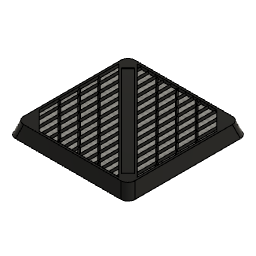
Air filter 120mm (Autodesk Fusion 360 design; units mm, degrees)
Autodesk Fusion 360 part; units mm, degrees
ref_plane "WorkPlane3" through (0, -60, 0) normal (0, 1, 0) x (0, 0, 1)
sketch "Frame bars" plane through (0, -60, 0) normal (0, 1, 0) x (1, 0, 0)
  line L0 (0, 0) -> (0, -95) construction
  line L1 (-60, 0) -> (-60, -25) construction
  line L2 (-52, 0) -> (-52, -10) construction
  line L3 (-44, 0) -> (-44, -10) construction
  line L4 (-36, 0) -> (-36, -10) construction
  line L5 (-28, 0) -> (-28, -10) construction
  line L6 (-20, 0) -> (-20, -10) construction
  line L7 (-12, 0) -> (-12, -10) construction
  line L8 (-4, 0) -> (-4, -10) construction
  line L9 (4, 0) -> (4, -10) construction
  line L10 (12, 0) -> (12, -10) construction
  line L11 (20, 0) -> (20, -10) construction
  line L12 (28, 0) -> (28, -10) construction
  line L13 (36, 0) -> (36, -10) construction
  line L14 (44, 0) -> (44, -10) construction
  line L15 (-63, -2) -> (49, -2) construction
  line L16 (0, 0) -> (49, 0) construction
  line L17 (-61, 0) -> (-60, -2)
  line L18 (-60, -2) -> (-59, 0)
  line L19 (-59, 0) -> (-61, 0)
  line L20 (-51, 0) -> (-53, 0)
  line L21 (-53, 0) -> (-52, -2)
  line L22 (-52, -2) -> (-51, 0)
  line L23 (-45, 0) -> (-44, -2)
  line L24 (-44, -2) -> (-43, 0)
  line L25 (-43, 0) -> (-45, 0)
  line L26 (-37, 0) -> (-36, -2)
  line L27 (-36, -2) -> (-35, 0)
  line L28 (-35, 0) -> (-37, 0)
  line L29 (-29, 0) -> (-28, -2)
  line L30 (-28, -2) -> (-27, 0)
  line L31 (-27, 0) -> (-29, 0)
  line L32 (-21, 0) -> (-20, -2)
  line L33 (-20, -2) -> (-19, 0)
  line L34 (-19, 0) -> (-21, 0)
  line L35 (-13, 0) -> (-12, -2)
  line L36 (-12, -2) -> (-11, 0)
  line L37 (-11, 0) -> (-13, 0)
  line L38 (-5, 0) -> (-4, -2)
  line L39 (-4, -2) -> (-3, 0)
  line L40 (-3, 0) -> (-5, 0)
  line L41 (3, 0) -> (4, -2)
  line L42 (4, -2) -> (5, 0)
  line L43 (11, 0) -> (12, -2)
  line L44 (12, -2) -> (13, 0)
  line L45 (20, -2) -> (21, 0)
  line L46 (19, 0) -> (20, -2)
  line L47 (28, -2) -> (29, 0)
  line L48 (27, 0) -> (28, -2)
  line L49 (36, -2) -> (37, 0)
  line L50 (35, 0) -> (36, -2)
  line L51 (44, -2) -> (45, 0)
  line L52 (43, 0) -> (44, -2)
  line L53 (5, 0) -> (3, 0)
  line L54 (13, 0) -> (11, 0)
  line L55 (21, 0) -> (19, 0)
  line L56 (29, 0) -> (27, 0)
  line L57 (37, 0) -> (35, 0)
  line L58 (45, 0) -> (43, 0)
  dimension "d1" = 60
  dimension "d2" = 8
  dimension "d3" = 8
  dimension "d4" = 8
  dimension "d5" = 8
  dimension "d6" = 8
  dimension "d7" = 8
  dimension "d8" = 8
  dimension "d9" = 8
  dimension "d10" = 8
  dimension "d11" = 8
  dimension "d12" = 8
  dimension "d13" = 8
  dimension "d14" = 8
  dimension "d15" = 2
  constraint coincident L0.start L16.start
  constraint vertical L0
  constraint vertical L1
  constraint vertical L2
  constraint vertical L3
  constraint vertical L4
  constraint vertical L5
  constraint vertical L6
  constraint vertical L7
  constraint vertical L8
  constraint vertical L9
  constraint vertical L10
  constraint vertical L11
  constraint vertical L12
  constraint parallel L12 L13
  constraint vertical L14
  constraint perpendicular L13 L15
  constraint perpendicular L14 L16
  constraint coincident L15 L17.end
  constraint coincident L1 L17.end
  constraint parallel L15 L19
  constraint perpendicular L2 L20
  constraint coincident L15 L21.end
  constraint coincident L2 L21.end
  constraint coincident L3 L23.end
  constraint coincident L15 L23.end
  constraint parallel L21 L23
  constraint parallel L22 L24
  constraint perpendicular L3 L25
  constraint coincident L4 L26.end
  constraint coincident L15 L26.end
  constraint parallel L24 L27
  constraint perpendicular L4 L28
  constraint coincident L15 L29.end
  constraint coincident L5 L29.end
  constraint parallel L27 L30
  constraint perpendicular L5 L31
  constraint coincident L6 L32.end
  constraint coincident L15 L32.end
  constraint parallel L30 L33
  constraint perpendicular L6 L34
  constraint coincident L7 L35.end
  constraint coincident L15 L35.end
  constraint parallel L33 L36
  constraint perpendicular L7 L37
  constraint coincident L8 L38.end
  constraint coincident L15 L38.end
  constraint parallel L36 L39
  constraint perpendicular L8 L40
  constraint coincident L16 L41.start
  constraint coincident L15 L41.end
  constraint parallel L38 L41
  constraint coincident L16 L42.end
  constraint parallel L39 L42
  constraint coincident L16 L43.start
  constraint coincident L15 L43.end
  constraint coincident L10 L43.end
  constraint coincident L16 L44.end
  constraint coincident L15 L45.start
  constraint coincident L11 L45.start
  constraint coincident L16 L45.end
  constraint coincident L16 L46.start
  constraint coincident L15 L47.start
  constraint coincident L12 L47.start
  constraint coincident L16 L47.end
  constraint parallel L45 L47
  constraint coincident L16 L48.start
  constraint parallel L46 L48
  constraint coincident L15 L49.start
  constraint coincident L13 L49.start
  constraint coincident L16 L49.end
  constraint parallel L47 L49
  constraint coincident L16 L50.start
  constraint parallel L48 L50
  constraint coincident L15 L51.start
  constraint coincident L14 L51.start
  constraint coincident L16 L51.end
  constraint parallel L49 L51
  constraint coincident L16 L52.start
  constraint parallel L50 L52
  measures "d1" distance of L0 L1
  measures "d2" distance of L1 L2
  measures "d3" distance of L2 L3
  measures "d4" distance of L3 L4
  measures "d5" distance of L4 L5
  measures "d6" distance of L5 L6
  measures "d7" distance of L6 L7
  measures "d8" distance of L7 L8
  measures "d9" distance of L8 L9
  measures "d10" distance of L9 L10
  measures "d11" distance of L10 L11
  measures "d12" distance of L11 L12
  measures "d13" distance of L12 L13
  measures "d14" distance of L13 L14
  measures "d15" distance of L15 L16
  measures "d95" distance of L0.start
  measures "d103" distance of L0.start
  measures "d104" distance of L0.start
sketch "Frame Edge" plane through (0, 0, 0) normal (0, 0, 1) x (1, 0, 0)
  line L0 (0, 0) -> (0, 72.5) construction
  line L1 (0, 0) -> (90, 0) construction
  circle A0 centre (-52.5, 52.5) radius 2.75
  circle A1 centre (-52.5, -52.5) radius 2.75
  circle A2 centre (52.5, 52.5) radius 2.75
  circle A3 centre (52.5, -52.5) radius 2.75
  line L2 (-57.4497, 47.5503) -> (47.5503, -57.4497)
  arc A4 (47.5503, -57.4497) -> (57.4497, -47.5503) centre (52.5, -52.5) ccw
  line L3 (57.4497, -47.5503) -> (-47.5503, 57.4497)
  arc A5 (-47.5503, 57.4497) -> (-57.4497, 47.5503) centre (-52.5, 52.5) ccw
  line L4 (-52.5, 52.5) -> (52.5, -52.5) construction
  circle A6 centre (-52.5, -52.5) radius 7
  circle A7 centre (52.5, 52.5) radius 7
  line L5 (59.5, 52.5) -> (59.5, -52.5)
  line L6 (-59.5, 52.5) -> (-59.5, -52.5)
  line L7 (52.5, 59.5) -> (-52.5, 59.5)
  line L8 (52.5, -59.5) -> (-52.5, -59.5)
  line L9 (35.5, 59.5) -> (59.5, 35.5)
  line L10 (35.5, 59.5) -> (69.5744, 59.5) construction
  line L11 (-59.5, -35.5) -> (-35.5, -59.5)
  line L12 (-52.5, 57.5) -> (52.5, 57.5)
  line L13 (-53.8563, -57.5) -> (52.5, -57.5)
  line L14 (-53.9142, 44.0147) -> (-52.5, 45.4289) construction
  line L15 (-52.5, 45.4289) -> (-44.0147, 53.9142) construction
  line L16 (44.0147, -53.9142) -> (53.9142, -44.0147) construction
  line L17 (-52.5, 45.4289) -> (45.4289, -52.5)
  line L18 (45.4289, -52.5) -> (52.5, -45.4289)
  line L19 (52.5, -45.4289) -> (-45.4289, 52.5)
  line L20 (-45.4289, 52.5) -> (-52.5, 45.4289)
  line L21 (-57.5, -52.5) -> (-57.5, 52.5)
  line L22 (57.5, -52.5) -> (57.5, 52.5)
  circle A8 centre (-52.5, -52.5) radius 5
  circle A9 centre (-52.5, 52.5) radius 5
  circle A10 centre (52.5, -52.5) radius 5
  circle A11 centre (52.5, 52.5) radius 5
  circle A12 centre (-52.5, 52.5) radius 4
  circle A13 centre (-52.5, -52.5) radius 4
  circle A14 centre (52.5, 52.5) radius 4
  circle A15 centre (52.5, -52.5) radius 4
  dimension "d19" = 5.5
  dimension "d20" = 52.5
  dimension "d21" = 52.5
  dimension "d22" = 14
  dimension "d23" = 14
  dimension "d24" = 14
  dimension "d25" = 45
  dimension "d26" = 24
  dimension "d27" = 2
  dimension "d28" = 2
  dimension "d29" = 5
  dimension "d30" = 5
  dimension "d31" = 2
  dimension "d32" = 2
  dimension "d33" = 2
  dimension "d117" = 10
  dimension "d118" = 8
  constraint coincident L0.start L1.start
  constraint vertical L0
  constraint perpendicular L0 L1
  constraint symmetric L1 A0 A1
  constraint symmetric L0 A0 A2
  constraint symmetric L0 A1 A3
  constraint tangent L2 A4
  constraint tangent A4 L3
  constraint parallel L2 L3
  constraint tangent L3 A5
  constraint tangent L2 A5
  constraint coincident A3.centre A4.centre
  constraint coincident A0.centre A5.centre
  constraint concentric A1 A6
  constraint concentric A2 A7
  constraint coincident A7 L5.start
  constraint coincident A4 L5.end
  constraint tangent A4 L5
  constraint tangent A7 L5
  constraint symmetric L0 L5.start L6.start
  constraint symmetric L0 L5.end L6.end
  constraint coincident A7 L7.start
  constraint coincident A5 L7.end
  constraint tangent A5 L7
  constraint tangent A7 L7
  constraint symmetric L1 L7.start L8.start
  constraint symmetric L1 L7.end L8.end
  constraint horizontal L10
  constraint coincident L7 L9.start
  constraint coincident L5 L9.end
  constraint symmetric L4 L9.start L11.start
  constraint symmetric L4 L9.end L11.end
  constraint perpendicular L0 L12
  constraint horizontal L13
  constraint perpendicular L4 L14
  constraint perpendicular L4 L15
  constraint perpendicular L4 L16
  constraint coincident L3 L16.end
  constraint coincident L2 L16.start
  constraint coincident L3 L15.end
  constraint coincident L2 L14.start
  constraint perpendicular L17 L18
  constraint parallel L17 L19
  constraint parallel L18 L20
  constraint coincident L16 L17.end
  constraint perpendicular L16 L17
  constraint vertical L21
  constraint symmetric L0 L21.start L22.start
  constraint symmetric L0 L21.end L22.end
  constraint concentric A1 A8
  constraint symmetric L1 A8 A9
  constraint symmetric L0 A8 A10
  constraint symmetric L0 A9 A11
  constraint coincident L13.end A10
  constraint coincident L21.start A8
  constraint coincident L21.end A9
  constraint coincident L12.start A9
  constraint coincident L12.end A11
  constraint concentric A0 A12
  constraint symmetric L1 A12 A13
  constraint symmetric L0 A12 A14
  constraint symmetric L0 A13 A15
  measures "d19" diameter of A0
  measures "d20" distance of L0 A0.centre
  measures "d21" distance of L1 A0.centre
  measures "d22" diameter of A4
  measures "d23" diameter of A6
  measures "d24" diameter of A7
  measures "d25" angle of L9 L10
  measures "d26" distance of L5 L9.start
  measures "d27" distance of L7 L12
  measures "d28" distance of L8 L13
  measures "d29" distance of A0.centre L15
  measures "d30" distance of A3.centre L16
  measures "d31" distance of L2 L17
  measures "d32" distance of L3 L19
  measures "d33" distance of L6 L21
  measures "d117" diameter of A8
  measures "d118" diameter of A12
extrude "Extrude1" add sketch "Frame Edge" along normal blind 3 contours L2 A4 A5 L13 L17 L18 L20 L21 A9 A10 | A5 L6 L11 L21 | A5 L12 L21 A9 | A4 L13 L22 A10 | A4 L8 L11 L13 | A6 L6 L11 L21 | A6 L11 L13 L21 | A9 | A6 L8 L11 L13 | A10 | A5 L7 L9 L12 | A6 L13 L21 A8 | A6 L13 L21 A8 | A4 L3 A5 L12 L18 L19 L20 L22 A9 A10 | A4 L5 L9 L22 | A7 L7 L9 L12 | A8 | A7 L5 L9 L22 | A7 L9 L12 L22 | A7 L12 L22 A11 | A7 L12 L22 A11 | A11 | A12 | A13 | A14 | A15 makes body 1
extrude "Extrude2" add sketch "Frame Edge" along normal blind 2 contours L17 L18 L19 L20 bodies 1
extrude "Extrude3" add sketch "Frame bars" along normal blind 90.5 from surface at 13 separate body contours L20 L21 L22 makes body 2
extrude "Extrude4" add sketch "Frame bars" along normal blind 94 from surface at 1.5 separate body contours L23 L24 L25 makes body 3
extrude "Extrude5" add sketch "Frame bars" along normal blind 86 from surface at 1.5 separate body contours L26 L27 L28 makes body 4
extrude "Extrude6" add sketch "Frame bars" along normal blind 78 from surface at 1.5 separate body contours L29 L30 L31 makes body 5
extrude "Extrude7" add sketch "Frame bars" along normal blind 70 from surface at 1.5 separate body contours L32 L33 L34 makes body 6
extrude "Extrude8" add sketch "Frame bars" along normal blind 62 from surface at 1.5 separate body contours L35 L36 L37 makes body 7
extrude "Extrude9" add sketch "Frame bars" along normal blind 54 from surface at 1.5 separate body contours L38 L39 L40 makes body 8
extrude "Extrude10" add sketch "Frame bars" along normal blind 46 from surface at 1.5 separate body contours L41 L42 L53 makes body 9
extrude "Extrude11" add sketch "Frame bars" along normal blind 38 from surface at 1.5 separate body contours L43 L44 L54 makes body 10
extrude "Extrude12" add sketch "Frame bars" along normal blind 30 from surface at 1.5 separate body contours L45 L46 L55 makes body 11
extrude "Extrude13" add sketch "Frame bars" along normal blind 22 from surface at 1.5 separate body contours L47 L48 L56 makes body 12
extrude "Extrude14" add sketch "Frame bars" along normal blind 14 from surface at 1.5 separate body contours L49 L50 L57 makes body 13
extrude "Extrude15" add sketch "Frame bars" along normal blind 6 from surface at 1.5 separate body contours L51 L52 L58 makes body 14
copy_body "CopyPasteBodies1" bodies 2 5 4 3 7 12 14 9 13 6 10 8 11 makes body 15 makes body 16 makes body 17 makes body 18 makes body 19 makes body 20 makes body 21 makes body 22 makes body 23 makes body 24 makes body 25 makes body 26 makes body 27
move_body "Move1" bodies 15 16 17 18 19 20 21 22 23 24 25 26 27 to x (-1, 0, 0) y (0, -1, 0) z (0, 0, 1) at (-0.0001, 0, 0)
combine "Combine1" operation add target body 1 tool bodies 5 4 2 3 15 22 20 24 23 25 26 17 16 19 21 18 7 12 14 9 13 6 10 8 11 27
extrude "Extrude16" add sketch "Frame Edge" along normal blind 3 contours A0 | A1 | A2 | A3 bodies 1
move_body "Move3" bodies 1 to x (1, 0, 0) y (0, 1, 0) z (0, 0, 1) at (0, 0, 50)
ref_plane "WorkPlane4" through (0, 0, 12.125) normal (-0.707107, 0.707107, 0) x (0, 0, 1)
sketch "Frame diagonal bars" plane through (0, 0, 12.125) normal (-0.707107, 0.707107, 0) x (0, 0, 1)
  line L0 (11, 0) -> (-19, 0) construction
  line L1 (-12.13, -82) -> (-12.13, -14) construction
  line L2 (-12.13, -14) -> (-12.13, 80) construction
  line L3 (-14, -67) -> (2, -67) construction
  line L4 (-14, -52) -> (2, -52) construction
  line L5 (-14, -37) -> (2, -37) construction
  line L6 (-14, -22) -> (2, -22) construction
  line L7 (-10.13, -82) -> (-10.13, -19)
  line L8 (-12.13, -66) -> (-12.13, -68)
  line L9 (-12.13, -53) -> (-10.13, -52)
  line L10 (-10.13, -52) -> (-12.13, -51)
  line L11 (-12.13, -51) -> (-12.13, -53)
  line L12 (-12.13, -38) -> (-10.13, -37)
  line L13 (-12.13, -23) -> (-10.13, -22)
  line L14 (-10.13, -22) -> (-12.13, -21)
  line L15 (-12.13, -21) -> (-12.13, -23)
  line L16 (-10.13, -37) -> (-12.13, -36)
  line L17 (-12.13, -36) -> (-12.13, -38)
  line L18 (-10.13, 52) -> (-12.13, 51)
  line L19 (-12.13, 53) -> (-10.13, 52)
  line L20 (-12.13, 51) -> (-12.13, 53)
  line L21 (-12.13, 66) -> (-10.13, 67)
  line L22 (-12.13, 68) -> (-10.13, 67)
  line L23 (-12.13, 66) -> (-12.13, 68)
  line L24 (-12.13, 38) -> (-10.13, 37)
  line L25 (-10.13, 37) -> (-12.13, 36)
  line L26 (-12.13, 36) -> (-12.13, 38)
  line L27 (-12.13, 23) -> (-10.13, 22)
  line L28 (-10.13, 22) -> (-12.13, 21)
  line L29 (-12.13, 21) -> (-12.13, 23)
  dimension "d90" = 12.13
  dimension "d92" = 67
  dimension "d93" = 15
  dimension "d94" = 15
  dimension "d95" = 15
  dimension "d96" = 2
  dimension "d98" = 1
  dimension "d99" = 1
  dimension "d100" = 1
  dimension "d101" = 1
  dimension "d103" = 1
  dimension "d104" = 1
  dimension "d105" = 1
  constraint horizontal L0
  constraint vertical L1
  constraint parallel L1 L2
  constraint perpendicular L1 L3
  constraint perpendicular L1 L4
  constraint perpendicular L1 L5
  constraint perpendicular L1 L6
  constraint perpendicular L5 L7
  constraint coincident L1 L8.end
  constraint coincident L1 L8.start
  constraint coincident L1 L9.start
  constraint coincident L4 L9.end
  constraint coincident L7 L9.end
  constraint coincident L1 L10.end
  constraint coincident L1 L12.start
  constraint coincident L5 L12.end
  constraint coincident L7 L12.end
  constraint coincident L1 L13.start
  constraint coincident L7 L13.end
  constraint coincident L6 L13.end
  constraint coincident L1 L14.end
  constraint coincident L1 L16.end
  constraint symmetric L0 L8.end L22.start
  constraint symmetric L0 L8.start L21.start
  constraint symmetric L0 L9.start L19.start
  constraint symmetric L0 L9.end L18.start
  constraint symmetric L0 L10.end L18.end
  constraint symmetric L0 L12.start L24.start
  constraint symmetric L0 L12.end L24.end
  constraint symmetric L0 L13.start L27.start
  constraint symmetric L0 L13.end L27.end
  constraint symmetric L0 L14.end L28.end
  constraint symmetric L0 L16.end L25.end
  measures "d90" distance of origin L2
  measures "d92" vertical distance of origin L3.end
  measures "d93" distance of L3 L4
  measures "d94" distance of L4 L5
  measures "d95" distance of L5 L6
  measures "d96" distance of L1 L7
  measures "d98" distance of L3 L8.end
  measures "d99" distance of L4 L9.start
  measures "d100" distance of L4 L10.end
  measures "d101" distance of L5 L12.start
  measures "d103" distance of L6 L13.start
  measures "d104" distance of L6 L14.end
  measures "d105" distance of L5 L16.end
move_body "Move5" bodies 1 to x (1, 0, 0) y (0, 1, 0) z (0, 0, 1) at (0, 0, -50)
extrude "Extrude17" add sketch "Frame diagonal bars" along normal mid plane 62 contours L9 L10 L11 | L18 L19 L20 bodies 1
extrude "Extrude19" add sketch "Frame diagonal bars" along normal mid plane 92 contours L12 L16 L17 | L24 L25 L26 bodies 1
extrude "Extrude20" add sketch "Frame diagonal bars" along normal mid plane 122 contours L13 L14 L15 | L27 L28 L29 bodies 1
copy_body "CopyPasteBodies3" bodies 1 makes body 28
move_body "Move6" bodies 28 to x (1, 0, 0) y (0, 1, 0) z (0, 0, 1) at (0, 0, 14)
extrude "Extrude21" cut sketch "Frame Edge" along normal through all contours A0 | A1 | A2 | A3 bodies 1
extrude "Extrude22" add sketch "Frame Edge" against normal blind 4 contours A12 | A13 | A14 | A15 bodies 1
sketch "Walls" plane through (0, 0, 0) normal (0, 0, 1) x (1, 0, 0)
  line L0 (59.5, -59.5) -> (-59.5, -59.5)
  line L1 (-59.5, -59.5) -> (-59.5, 59.5)
  line L2 (-59.5, 59.5) -> (59.5, 59.5)
  line L3 (59.5, 59.5) -> (59.5, -59.5)
  line L4 (59.5, -59.5) -> (-59.5, 59.5) construction
  line L5 (-59.5, -59.5) -> (59.5, 59.5) construction
  line L6 (57.5, 57.5) -> (-57.5, 57.5)
  line L7 (-57.5, 57.5) -> (-57.5, -57.5)
  line L8 (-57.5, -57.5) -> (57.5, -57.5)
  line L9 (57.5, -57.5) -> (57.5, 57.5)
  line L10 (57.5, 57.5) -> (-57.5, -57.5) construction
  line L11 (-57.5, 57.5) -> (57.5, -57.5) construction
  line L12 (-64, 64) -> (64, 64)
  line L13 (64, 64) -> (64, -64)
  line L14 (64, -64) -> (-64, -64)
  line L15 (-64, -64) -> (-64, 64)
  line L16 (-64, 64) -> (64, -64) construction
  line L17 (64, 64) -> (-64, -64) construction
  line L18 (62, 62) -> (-62, 62)
  line L19 (-62, 62) -> (-62, -62)
  line L20 (-62, -62) -> (62, -62)
  line L21 (62, -62) -> (62, 62)
  line L22 (62, 62) -> (-62, -62) construction
  line L23 (-62, 62) -> (62, -62) construction
  dimension "d128" = 119
  dimension "d129" = 119
  dimension "d130" = 2
  dimension "d131" = 4.5
  dimension "d132" = 2
  dimension "d134" = 2
  dimension "d135" = 4.5
  constraint perpendicular L0 L1
  constraint parallel L0 L2
  constraint parallel L1 L3
  constraint horizontal L0
  constraint coincident L4 origin
  constraint coincident L5 origin
  constraint perpendicular L6 L7
  constraint parallel L6 L8
  constraint parallel L7 L9
  constraint horizontal L6
  constraint coincident L5 L6.start
  constraint coincident L10 origin
  constraint coincident L11 origin
  constraint perpendicular L12 L13
  constraint parallel L12 L14
  constraint parallel L13 L15
  constraint horizontal L12
  constraint coincident L16 origin
  constraint coincident L17 origin
  constraint perpendicular L18 L19
  constraint parallel L18 L20
  constraint parallel L19 L21
  constraint horizontal L18
  constraint coincident L17 L18.start
  constraint coincident L22 origin
  constraint coincident L23 origin
  measures "d128" distance of L1.end L2.end
  measures "d129" distance of L0.end L1.end
  measures "d130" distance of L2 L6
  measures "d131" distance of L2 L12
  measures "d132" distance of L12 L18
  measures "d134" distance of L15 L19
  measures "d135" distance of L1 L15
extrude "Extrude26" add sketch "Walls" along normal blind 13 draft -18.435 separate body contours L0 L1 L2 L3 | L6 L7 L8 L9 | L12 L13 L14 L15 | L18 L19 L20 L21 makes body 29
extrude "Extrude27" cut sketch "Walls" along normal blind 13 draft -18.435 contours L0 L1 L2 L3 | L6 L7 L8 L9 | L18 L19 L20 L21 bodies 29
copy_body "CopyPasteBodies4" bodies 29 makes body 30
move_body "Move7" bodies 30 to x (1, 0, 0) y (0, 1, 0) z (0, 0, 1) at (0, 0, 4)
extrude "Extrude28" cut sketch "Walls" along normal blind 4 contours L0 L1 L2 L3 | L6 L7 L8 L9 | L12 L13 L14 L15 | L18 L19 L20 L21 bodies 29
extrude "Extrude29" cut sketch "Walls" against normal blind 3 from surface at 13 contours L0 L1 L2 L3 | L6 L7 L8 L9 | L12 L13 L14 L15 | L18 L19 L20 L21 bodies 29
move_body "Move8" bodies 29 to x (1, 0, 0) y (0, 1, 0) z (0, 0, 1) at (0, 0, -7)
fillet "Fillet1" radius 8 8 edges at (-61.6667, -61.6667, 0) (-59.6667, -59.6667, 0) (61.6667, 61.6667, 0) (59.6667, 59.6667, 0) (61.6667, -61.6667, 0) (59.6667, -59.6667, 0) (-61.6667, 61.6667, 0) (-59.6667, 59.6667, 0) on bodies 29
combine "Combine2" operation add target body 1 tool bodies 29
fillet "Fillet2" radius 8 8 edges at (61.8333, -61.8333, 10.5) (59.8333, -59.8333, 10.5) (-61.8333, 61.8333, 10.5) (-59.8333, 59.8333, 10.5) (-61.8333, -61.8333, 10.5) (-59.8333, -59.8333, 10.5) (61.8333, 61.8333, 10.5) (59.8333, 59.8333, 10.5) on bodies 30
combine "Combine3" operation add target body 28 tool bodies 30
move_body "Move9" bodies 28 to x (1, 0, 0) y (0, 1, 0) z (0, 0, 1) at (0, 0, -7)
sketch "Filter" plane through (0, 0, 3) normal (0, 0, 1) x (-1, 0, 0)
  ellipse E0 centre (52.2339, -52.2339) end of major axis (58.4878, -58.4878) minor radius 8 (53.0772, -60.6667) -> (60.6667, -53.0772) ccw
  line L0 (60.6667, -53.0772) -> (60.6667, 53.0772)
  ellipse E1 centre (52.2339, 52.2339) end of major axis (58.4878, 58.4878) minor radius 8 (60.6667, 53.0772) -> (53.0772, 60.6667) ccw
  line L1 (53.0772, 60.6667) -> (-53.0772, 60.6667)
  ellipse E2 centre (-52.2339, 52.2339) end of major axis (-58.4878, 58.4878) minor radius 8 (-53.0772, 60.6667) -> (-60.6667, 53.0772) ccw
  line L2 (-60.6667, 53.0772) -> (-60.6667, -53.0772)
  ellipse E3 centre (-52.2339, -52.2339) end of major axis (-58.4878, -58.4878) minor radius 8 (-60.6667, -53.0772) -> (-53.0772, -60.6667) ccw
  line L3 (-53.0772, -60.6667) -> (53.0772, -60.6667)
  circle A0 centre (52.5, -52.5) radius 2.75
  circle A1 centre (-52.5, -52.5) radius 2.75
  circle A2 centre (52.5, 52.5) radius 2.75
  circle A3 centre (-52.5, 52.5) radius 2.75
  line L4 (57.5, 37.5) -> (57.5, -47.601)
  arc A4 (57.5, -47.601) -> (57.4497, -47.5503) centre (52.5, -52.5) ccw
  line L5 (57.4497, -47.5503) -> (-47.5503, 57.4497)
  arc A5 (-47.5503, 57.4497) -> (-47.601, 57.5) centre (-52.5, 52.5) ccw
  line L6 (-47.601, 57.5) -> (37.5, 57.5)
  line L7 (37.5, 57.5) -> (57.5, 37.5)
  line L8 (52.5, -45.4289) -> (45.4289, -52.5)
  line L9 (45.4289, -52.5) -> (-52.5, 45.4289)
  line L10 (-52.5, 45.4289) -> (-45.4289, 52.5)
  line L11 (-45.4289, 52.5) -> (52.5, -45.4289)
  line L12 (-57.5, -37.5) -> (-57.5, 47.601)
  arc A6 (-57.5, 47.601) -> (-57.4497, 47.5503) centre (-52.5, 52.5) ccw
  line L13 (-57.4497, 47.5503) -> (47.5503, -57.4497)
  arc A7 (47.5503, -57.4497) -> (47.601, -57.5) centre (52.5, -52.5) ccw
  line L14 (47.601, -57.5) -> (-37.5, -57.5)
  line L15 (-37.5, -57.5) -> (-57.5, -37.5)
  line L16 (-58.5, -58.5) -> (58.5, -58.5)
  line L17 (58.5, -58.5) -> (58.5, 58.5)
  line L18 (58.5, 58.5) -> (-58.5, 58.5)
  line L19 (-58.5, 58.5) -> (-58.5, -58.5)
  line L20 (-58.5, -58.5) -> (58.5, 58.5) construction
  line L21 (58.5, -58.5) -> (-58.5, 58.5) construction
  dimension "d162" = 117
  dimension "d163" = 117
  constraint perpendicular L16 L17
  constraint parallel L16 L18
  constraint parallel L17 L19
  constraint horizontal L16
  constraint coincident L20 origin
  constraint coincident L21 origin
  measures "d162" distance of L17.end L18.end
  measures "d163" distance of L16.end L17.end
extrude "Extrude30" add sketch "Filter" along normal blind 2 from surface at 1 separate body contours E0 E1 E2 E3 L16 L17 L18 L19 | A0 | A1 | A2 | A3 | L4 A4 L5 A5 L6 L7 | L8 L9 L10 L11 | L12 A6 L13 A7 L14 L15 makes body 31
equation "d3 = d2"
equation "d4 = d2"
equation "d5 = d2"
equation "d6 = d2"
equation "d7 = d2"
equation "d8 = d2"
equation "d9 = d2"
equation "d10 = d2"
equation "d11 = d2"
equation "d12 = d2"
equation "d13 = d2"
equation "d14 = d2"
equation "d23 = d22"
equation "d24 = d22"
equation "d92 = ( 134 / 2 ) * 1 mm"
equation "d94 = d93"
equation "d95 = d93"
equation "d99 = d98"
equation "d100 = d99"
equation "d101 = d98"
equation "d103 = d98"
equation "d104 = d103"
equation "d105 = d101"
equation "d117 = d23 - d28 * 2"
equation "d128 = d20 * 2 + d22"
equation "d129 = d21 * 2 + d22"
equation "d132 = d130"
equation "d134 = d132"
equation "d135 = d131"
named bodies: "Inner Frame", "Inner Frame grid", "Outer Frame", "Inner frame walls", "Outer frame walls"
